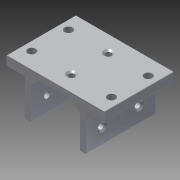
# Autodesk Inventor part: 6835_p
Saved by Autodesk Inventor 2013 (Build 170138000, 138)
## iProperties
Category: PARTsolutions
Company: 8020
Created: 2013-09-15
Part Number: 6835_p
Catalog Web Link: www.cadenas.de
Description: 6835, 6535, 6836, 6536_p-High-Cycle Double Flange Linear Bearings
Vendor: 8020
Document SubType Name: Modeling
Designer: PARTuser1
Manufacturer: 8020
Density: 2.71 g/cm^3
Material: Aluminum 6061
Mass: 252.741 g
Surface Area: 298.984 cm^2
Volume: 93.2625 cm^3
PSOL_IDENT_0: {$CADENAS_DATA\23d-libs\8020\inch\linear_motion\6835.prj},167 {VTYP=3D},{NB=6835_p},{LINA=6835_p},{N
PSOL_IDENT_1: N=6835, 6535, 6836, 6536_p},{DATE=22.08.2012},{GEOMDATE=03.02.2012 00:00:00},{VERSION=},{LINEID=10},
PSOL_IDENT_2: {LINESUBID=-1},{WBVAR=TS,N}  {NB=6835_p},{LINA=6835_p},{KT=DUMMY},{PN=6835},{TS=0},{A=1.500},{B=0.50
PSOL_IDENT_3: 0},{C=2.500},{D=0.625},{E=1.250},{F=0.375},{G=4.000},{H=0.750},{J=3.250},{K=1.250},{L=1.875},{M=1.50
PSOL_IDENT_4: 0},{N=2.812},{P=0.656},{Q=0.000},{R=0.375},{S=0.125},{T=0.328},{W=.665},{TH=0.250},{CD=0.385},{CHD=0
PSOL_IDENT_5: .245},{CDPTH=0.0588},{PC=White},{BR=1},{BHD=0.344},{ST=3628}
CNS_NT: High-Cycle Double Flange Linear Bearings
CNS_NB: 6835_p
CNS_NBSYN: $PN._p
CNS_LINA: 6835_p
CNS_PN: 6835
CNS_TS: w/o Pre-drilled Brake Holes
CNS_A: 1.500
CNS_B: 0.500
CNS_C: 2.500
CNS_D: 0.625
CNS_E: 1.250
CNS_F: 0.375
CNS_G: 4.000
CNS_H: 0.750
CNS_J: 3.250
CNS_K: 1.250
CNS_L: 1.875
CNS_M: 1.500
CNS_N: 2.812
CNS_P: 0.656
CNS_Q: 0.000
CNS_R: 0.375
CNS_S: 0.125
CNS_T: 0.328
CNS_W: .665
CNS_TH: 0.250
CNS_CD: 0.385
CNS_CHD: 0.245
CNS_CDPTH: 0.0588
CNS_PC: White
CNS_BR: 1
CNS_BHD: 0.344
CNS_ST: 3628
SUPPLIER: 8020
ARTICLENO: 6835_p
BOMINFO: 6835_p
CREATOR: CADENAS GmbH
Title: 6835_p
Author: Cadenas PARTsolutions
Comments: High-Cycle Double Flange Linear Bearings
Autodesk Inventor part; units mm, degrees
sketch "Sketch_1" plane through (0, 0, 0) normal (0, 0, 1) x (1, 0, 0)
  line L0 (-50.8, 30.988) -> (-50.8, 22.987)
  arc A0 (-50.8, 22.987) -> (-50.038, 22.225) centre (-50.038, 22.987) ccw
  line L1 (-50.038, 22.225) -> (-32.512, 22.225)
  arc A1 (-31.75, 21.463) -> (-32.512, 22.225) centre (-32.512, 21.463) ccw
  line L2 (-31.75, 21.463) -> (-31.75, -15.113)
  arc A2 (-31.75, -15.113) -> (-30.988, -15.875) centre (-30.988, -15.113) ccw
  line L3 (-30.988, -15.875) -> (-26.162, -15.875)
  arc A3 (-26.162, -15.875) -> (-25.4, -15.113) centre (-26.162, -15.113) ccw
  line L4 (-25.4, -15.113) -> (-25.4, 17.4498)
  line L5 (-25.4, 17.4498) -> (-17.4498, 25.4)
  line L6 (-17.4498, 25.4) -> (17.4498, 25.4)
  line L7 (17.4498, 25.4) -> (25.4, 17.4498)
  line L8 (25.4, 17.4498) -> (25.4, -15.113)
  arc A4 (25.4, -15.113) -> (26.162, -15.875) centre (26.162, -15.113) ccw
  line L9 (26.162, -15.875) -> (30.988, -15.875)
  arc A5 (30.988, -15.875) -> (31.75, -15.113) centre (30.988, -15.113) ccw
  line L10 (31.75, -15.113) -> (31.75, 21.463)
  arc A6 (32.512, 22.225) -> (31.75, 21.463) centre (32.512, 21.463) ccw
  line L11 (32.512, 22.225) -> (50.038, 22.225)
  arc A7 (50.038, 22.225) -> (50.8, 22.987) centre (50.038, 22.987) ccw
  line L12 (50.8, 22.987) -> (50.8, 30.988)
  arc A8 (50.8, 30.988) -> (50.038, 31.75) centre (50.038, 30.988) ccw
  line L13 (50.038, 31.75) -> (-50.038, 31.75)
  arc A9 (-50.038, 31.75) -> (-50.8, 30.988) centre (-50.038, 30.988) ccw
  constraints: 28 end point, 20 point on circle, 10 centre point
extrude "Extrusion1" add sketch "Sketch_1" along normal mid plane 71.4248
sketch "Sketch2" plane through (31.75, -15.113, 35.7124) normal (1, 0, 0) x (0, 0, -1)
  point P0 (16.6624, 15.113)
hole "Drilling 1" at (31.75, 0, 19.05) direction (-1, 0, 0) diameter 6.223 depth 63.5 countersink diameter 9.779 countersink angle 99.939
pattern_linear "Rectangular Pattern1" count 2 spacing 38.1 along (0, 0, -1) of "Drilling 1"
sketch "Sketch3" plane through (-50.038, 31.75, 35.7124) normal (0, 1, 0) x (1, 0, 0)
  point P0 (50.038, 16.6624)
hole "Drilling 2" at (0, 31.75, 19.05) direction (0, -1, 0) diameter 6.223 depth 6.35 countersink diameter 9.779 countersink angle 99.939
pattern_linear "Rectangular Pattern2" count 2 spacing 38.1 along (0, 0, -1) of "Drilling 2"
sketch "Sketch4" plane through (-50.038, 31.75, 35.7124) normal (0, 1, 0) x (1, 0, 0)
  point P0 (8.763, 16.6624)
hole "Drilling 3" at (-41.275, 31.75, 19.05) direction (0, -1, 0) diameter 8.3312 depth 9.525
pattern_linear "Rectangular Pattern3" count 2 spacing 82.55 along (1, 0, 0) count 2 spacing 38.1 along (0, 0, -1) of "Drilling 3"
ref_plane "pad1_XY" through (-25.4, 0, 19.05) normal (1, 0, 0) x (0, 0, -1)
ref_plane "pad1_YZ" through (-25.4, 0, 19.05) normal (0, 0, -1) x (0, 1, 0)
ref_plane "pad1_ZX" through (-25.4, 0, 19.05) normal (0, 1, 0) x (1, 0, 0)
ref_plane "pad2_XY" through (25.4, 0, 19.05) normal (1, 0, 0) x (0, 0, -1)
ref_plane "pad2_YZ" through (25.4, 0, 19.05) normal (0, 0, -1) x (0, 1, 0)
ref_plane "pad2_ZX" through (25.4, 0, 19.05) normal (0, 1, 0) x (1, 0, 0)
ref_plane "pad3_XY" through (0, 25.4, 19.05) normal (0, 1, 0) x (1, 0, 0)
ref_plane "pad3_YZ" through (0, 25.4, 19.05) normal (1, 0, 0) x (0, 0, -1)
ref_plane "pad3_ZX" through (0, 25.4, 19.05) normal (0, 0, -1) x (0, 1, 0)
ref_plane "s1_1_XY" through (-30.2565, 0, 19.05) normal (1, 0, 0) x (0, 0, -1)
ref_plane "s1_1_YZ" through (-30.2565, 0, 19.05) normal (0, 0, -1) x (0, 1, 0)
ref_plane "s1_1_ZX" through (-30.2565, 0, 19.05) normal (0, 1, 0) x (1, 0, 0)
ref_plane "s1_2_XY" through (-30.2565, 0, -19.05) normal (1, 0, 0) x (0, 0, -1)
ref_plane "s1_2_YZ" through (-30.2565, 0, -19.05) normal (0, 0, -1) x (0, 1, 0)
ref_plane "s1_2_ZX" through (-30.2565, 0, -19.05) normal (0, 1, 0) x (1, 0, 0)
ref_plane "s2_1_XY" through (30.2565, 0, 19.05) normal (1, 0, 0) x (0, 0, -1)
ref_plane "s2_1_YZ" through (30.2565, 0, 19.05) normal (0, 0, -1) x (0, 1, 0)
ref_plane "s2_1_ZX" through (30.2565, 0, 19.05) normal (0, 1, 0) x (1, 0, 0)
ref_plane "s2_2_XY" through (30.2565, 0, -19.05) normal (1, 0, 0) x (0, 0, -1)
ref_plane "s2_2_YZ" through (30.2565, 0, -19.05) normal (0, 0, -1) x (0, 1, 0)
ref_plane "s2_2_ZX" through (30.2565, 0, -19.05) normal (0, 1, 0) x (1, 0, 0)
ref_plane "s3_1_XY" through (0, 30.2565, 19.05) normal (0, 1, 0) x (1, 0, 0)
ref_plane "s3_1_YZ" through (0, 30.2565, 19.05) normal (1, 0, 0) x (0, 0, -1)
ref_plane "s3_1_ZX" through (0, 30.2565, 19.05) normal (0, 0, -1) x (0, 1, 0)
ref_plane "s3_2_XY" through (0, 30.2565, -19.05) normal (0, 1, 0) x (1, 0, 0)
ref_plane "s3_2_YZ" through (0, 30.2565, -19.05) normal (1, 0, 0) x (0, 0, -1)
ref_plane "s3_2_ZX" through (0, 30.2565, -19.05) normal (0, 0, -1) x (0, 1, 0)
body "Solid1"
